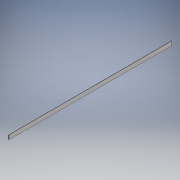
# Autodesk Inventor part: Boden_airline_rund
Saved by Autodesk Inventor 2018 (Build 220112000, 112)
## iProperties
Created: 2020-03-29
Part Number: Boden_airline_rund
Material: Generisch
Document SubType Name: Blech
Designer: wepet
Density: 1 g/cm^3
Sheet Metal Rule: Standard_mm
Appearance: Vorgabe
Author: wepet
Autodesk Inventor part; units mm, degrees
ref_plane "YZ Plane" through (0, 0, 0) normal (1, 0, 0) x (0, 1, 0)
ref_plane "XZ Plane" through (0, 0, 0) normal (0, 1, 0) x (-1, 0, 0)
ref_plane "XY Plane" through (0, 0, 0) normal (0, 0, 1) x (1, 0, 0)
sketch "Skizze2" plane through (0, 0, 0) normal (0, 1, 0) x (-1, 0, 0)
  line L0 (0, -5) -> (0, 0) construction
  line L1 (0.85, -4.7) -> (0.85, -0.3) construction
  line L2 (0.85, -0.3) -> (0.3, -0.3) construction
  line L3 (0.3, -0.3) -> (0.3, -4.7) construction
  line L4 (0.3, -4.7) -> (0.85, -4.7) construction
  line L5 (-0.0744, -2.5) -> (0, -2.5) construction
  line L6 (1.15, -3) -> (0.85, -3)
  line L7 (0, 0) -> (0, -5)
  line L8 (0.3, -4.7) -> (0.3, -0.3)
  line L9 (0.3, -4.7) -> (0.3, -5) construction
  line L10 (0.3, -0.3) -> (0.3, 0) construction
  line L11 (0.3, 0) -> (0, 0) construction
  line L12 (0.3, 0) -> (0, 0)
  line L13 (0.3, -5) -> (0, -5)
  line L14 (0, -2.5) -> (0.3, -2.5) construction
  ellipse E0 centre (0.3, -2.5) end of major axis (0.3, -5) minor radius 0.8675 (0.3, -5) -> (1.15, -3) ccw
  ellipse E1 centre (0.3, -2.5) end of major axis (0.3, -4.7) minor radius 0.5648 (0.3, -4.7) -> (0.85, -3) ccw
  line L15 (1.15, -2) -> (0.85, -2)
  line L16 (1.15, -3) -> (1.15, -2) construction
  ellipse E2 centre (0.3, -2.5) end of major axis (0.3, -0.3) minor radius 0.5648 (0.85, -2) -> (0.3, -0.3) ccw
  ellipse E3 centre (0.3, -2.5) end of major axis (0.3, 0) minor radius 0.8675 (1.15, -2) -> (0.3, 0) ccw
  dimension "d3" = 0.5
  dimension "d7" = 5
  dimension "d8" = 1.15
  dimension "d9" = 0.3
  dimension "d10" = 0.3
  dimension "d11" = 0.3
  dimension "d12" = 0.5
  constraints: 34 end point, 6 perpendicular, 5 vertical, 4 coincident, 4 point on line, 3 midpoint, 3 parallel, 2 collinear, 16 other
  measures "d3" distance between parallel lines of L6 L5
  measures "d7" distance between parallel lines of L11 L13
  measures "d8" distance from line of L0 L6.start
  measures "d9" distance between parallel lines of L0 L3
  measures "d10" distance of L6.start L6.end
  measures "d11" distance between parallel lines of L13 L4
  measures "d12" distance between parallel lines of L15 L14
extrude "Extrusion1" add sketch "Skizze2" along normal blind 197.5
equation "\"Biegeradius\" = Stärke"
equation "\"BreiteBiegungsfreistellung\" = Stärke"
equation "\"TiefeBiegungsfreistellung\" = 0.5 * Stärke"
equation "\"GrößeEckenfreistellung\" = 4 * Stärke"
equation "\"MinimalRest\" = 2 * Stärke"
equation "\"Übergangsradius\" = Biegeradius"
equation "\"JacobiRadiusGröße\" = Biegeradius"
equation "\"Abstandsgröße\" = Stärke"
equation "\"Stärke\" = 0.5"
